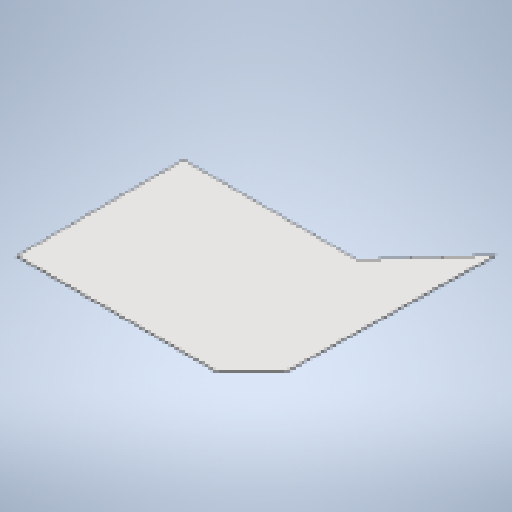
# Autodesk Inventor part: BSH 015 board cone 5
Saved by Autodesk Inventor 2025 (Build 290162010, 162A)
## iProperties
Created: 2024-07-23
Part Number: BSH 015 board cone 5
Material: 09g2s
Document SubType Name: Sheet Metal
Designer: admin
Mass: 40581.4 g
Surface Area: 34651.2 cm^2
Volume: 5169.6 cm^3
Density: 7.85 g/cm^3
Sheet Metal Rule: AISI304 3mm Die 32
Sheet Metal Width: 0,000 mm
Sheet Metal Length: 0,000 mm
Sheet Metal Area: 0,000 mm^2
Appearance: Default
Author: admin
Autodesk Inventor part; units mm, degrees
ref_plane "YZ Plane" through (0, 0, 0) normal (1, 0, 0) x (0, 1, 0)
ref_plane "XZ Plane" through (0, 0, 0) normal (0, 1, 0) x (-1, 0, 0)
ref_plane "XY Plane" through (0, 0, 0) normal (0, 0, 1) x (1, 0, 0)
sketch "Sketch8" plane through (0, 0, 0) normal (0, 0, 1) x (1, 0, 0)
  line L0 (0, 2897) -> (1200, 2897)
  line L1 (1200, 2897) -> (1200, 0)
  line L2 (1200, 0) -> (0, 0)
  line L3 (0, 0) -> (0, 2897)
  line L4 (0, 2897) -> (1200, 0) construction
  line L5 (1200, 2897) -> (0, 0) construction
  line L6 (947, 0) -> (1097, 150)
  line L7 (1097, 150) -> (1147, 2897)
  line L8 (0, 700) -> (1200, 700)
  line L9 (1112.5806, 1006) -> (837.057, 700)
  line L10 (110.253, 0) -> (110.253, 700)
  point P0 (600, 1448.5)
  point P1 (1107.0109, 700)
  dimension "d43" = 1200
  dimension "d44" = 2897
  dimension "d45" = 53
  dimension "d46" = 947
  dimension "d47" = 150
  dimension "d48" = 103
  dimension "d49" = 700
  dimension "d55" = 306
  dimension "d57" = 110.253
  dimension "d61" = 48
  measures "d43" distance of L1.end L2.end
  measures "d44" distance of L0.end L1.end
  measures "d45" distance of L0.end L7.end
  measures "d46" distance of point (0, 0) L6.start
  measures "d47" distance from line of L2 L6.end
  measures "d48" distance from line of L1 L6.end
  measures "d49" distance of L1.end L8.end
  measures "d55" distance from line of L8 L9.start
  measures "d57" distance between parallel lines of L3 L10
  measures "d61" angle of L8 L9
extrude "Plate4" add sketch "Sketch8" against normal blind 3 contours L7 L8 L9 | L8 L7 L6 L2 L10
chamfer "Corner Chamfer1" distance 6 angle 45 2 edges at (947, 0, -1.5) (1097, 150, -1.5)
equation "\"d50\" = Thickness"
equation "\"BendReliefWidth\" = Thickness"
equation "\"BendReliefDepth\" = 0.5 * Thickness"
equation "\"CornerReliefSize\" = 4 * Thickness"
equation "\"MinimumRemnant\" = 2 * Thickness"
equation "\"TransitionRadius\" = BendRadius"
equation "\"JacobiRadiusSize\" = BendRadius"
equation "\"GapSize\" = Thickness"
equation "\"Thickness\" = 3"
equation "\"BendRadius\" = 5"
body "Solid2"
